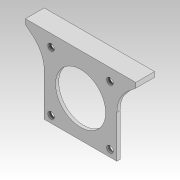
# Autodesk Inventor part: J2MotorBracket
Saved by Autodesk Inventor 2020 (Build 240168000, 168)
## iProperties
Created: 2021-11-21
Part Number: J2MotorBracket
Material: Generic
Document SubType Name: Modeling
Designer: DDeGo
Density: 1 g/cm^3
Appearance: Default
Author: DDeGo
Autodesk Inventor part; units mm, degrees
ref_plane "YZ Plane" through (0, 0, 0) normal (1, 0, 0) x (0, 1, 0)
ref_plane "XZ Plane" through (0, 0, 0) normal (0, 1, 0) x (-1, 0, 0)
ref_plane "XY Plane" through (0, 0, 0) normal (0, 0, 1) x (1, 0, 0)
sketch "Sketch1" plane through (0, 0, 0) normal (0, 0, 1) x (1, 0, 0)
  line L0 (-23.5, -23.5) -> (23.5, -23.5) construction
  line L1 (23.5, -23.5) -> (23.5, 23.5) construction
  line L2 (23.5, 23.5) -> (-23.5, 23.5) construction
  line L3 (-23.5, 23.5) -> (-23.5, -23.5) construction
  line L4 (-23.5, -23.5) -> (23.5, 23.5) construction
  line L5 (23.5, -23.5) -> (-23.5, 23.5) construction
  circle A0 centre (0, 0) radius 20
  circle A1 centre (-23.5, 23.5) radius 2.6
  circle A2 centre (23.5, 23.5) radius 2.6
  circle A3 centre (23.5, -23.5) radius 2.6
  circle A4 centre (-23.5, -23.5) radius 2.6
  line L6 (29, 29) -> (-29, 29)
  line L7 (-29, 29) -> (-29, -29)
  line L8 (-29, -29) -> (29, -29)
  line L9 (29, -29) -> (29, 29)
  line L10 (29, 29) -> (-29, -29) construction
  line L11 (-29, 29) -> (29, -29) construction
  dimension "d0" = 5.2
  dimension "d1" = 47
  dimension "d2" = 47
  dimension "d3" = 40
  dimension "d4" = 58
  constraints: 24 end point, 5 centre point, 5 coincident, 4 midpoint, 4 parallel, 3 equal radius, 2 horizontal, 2 perpendicular, 1 point on line
  measures "d0" diameter of A1
  measures "d1" distance of L1.end L2.end
  measures "d2" distance of L0.end L1.end
  measures "d3" diameter of A0
  measures "d4" distance of L6.start L6.end
extrude "Extrusion1" add sketch "Sketch1" along normal blind 2.5
sketch "Sketch2" plane through (-29, 29, 0) normal (0, 1, 0) x (1, 0, 0)
  line L0 (58, 0) -> (0, 0) construction
  line L1 (0, 0) -> (0, -2.5) construction
  line L2 (58, -2.5) -> (0, -2.5) projected
  line L3 (58, 0) -> (58, -2.5) construction
  line L4 (58, -2.5) -> (0, -2.5) projected
  line L5 (0, -2.5) -> (-15, -2.5)
  line L6 (-15, -2.5) -> (-15, 12.5)
  line L7 (-15, 12.5) -> (73, 12.5)
  line L8 (73, 12.5) -> (73, -2.5)
  line L9 (73, -2.5) -> (58, -2.5)
  point P0 (29, 0)
  dimension "d7" = 15
  dimension "d8" = 15
  constraints: 10 end point, 4 perpendicular, 1 collinear, 1 horizontal, 1 point on line
  measures "d7" distance of L1.end L5.end
  measures "d8" distance of L5.end L6.end
extrude "Extrusion2" add sketch "Sketch2" along normal blind 4
sketch "Sketch3" plane through (-44, 29, -12.5) normal (-1, 0, 0) x (0, 0, 1)
  line L0 (0, 0) -> (15, 0) projected
  line L1 (15, 0) -> (15, -58) construction
  line L2 (15, 0) -> (15, -12.5)
  line L3 (15, -12.5) -> (12.5, -12.5)
  line L4 (12.5, -12.5) -> (0, 0)
  line L5 (12.5, 0) -> (15, 0) projected
  point P0 (12.5, -29)
  dimension "d20" = 45
  constraints: 6 end point, 1 horizontal, 1 parallel, 1 point on line, 1 vertical
  measures "d20" angle of L0 L4
extrude "Extrusion3" add sketch "Sketch3" against normal up to surface (15 mm away)
sketch "Sketch4" plane through (0, 0, 2.5) normal (0, 0, 1) x (1, 0, 0)
  line L0 (-29, 16.5) -> (-44, 29)
  line L1 (-44, 16.5) -> (-44, 33) construction
  line L2 (-44, 29) -> (-44, 16.5)
  line L3 (-44, 16.5) -> (-29, 16.5) projected
  point P0 (0, 0)
  constraints: 4 end point, 1 coincident, 1 point on line, 1 vertical
extrude "Extrusion4" cut sketch "Sketch4" against normal through all
mirror "Mirror1" about plane through (0, 0, 0) normal (1, 0, 0) of "Extrusion3", "Extrusion4"
fillet "Fillet1" radius 25 2 edges at (-29, 16.5, 1.25) (29, 16.5, 1.25)
body "Solid1"
